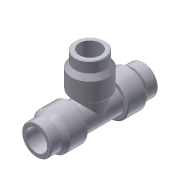
# Autodesk Inventor part: 0pvc_T_0.75
Saved by Autodesk Inventor 2016 (Build 200138000, 138)
## iProperties
Company: HERA Project
Created: 2013-06-12
Part Number: 0pvc_T_0.75
Material: PVC-Piping
Document SubType Name: Modeling
Designer: David DeBoer
Density: 1.4 g/cm^3
Description: 3/4" PVC Tee
Mass: 47.0427 g
Surface Area: 211.064 cm^2
Volume: 33.6019 cm^3
Appearance: Smooth - White
Author: David DeBoer
Title: PVC-T-0.75
Autodesk Inventor part; units mm, degrees
sketch "Sketch1" plane through (0, 0, 0) normal (0, 0, 1) x (1, 0, 0)
  circle A0 centre (0, 0) radius 14.5
  dimension "d0" = 29
  constraints: 1 centre point, 1 coincident
  measures "d0" diameter of A0
extrude "mainBody" add sketch "Sketch1" along normal mid plane 111
sketch "Sketch10" plane through (0, 0, 55.5) normal (0, 0, 1) x (1, 0, 0)
  circle A0 centre (0, 0) radius 30.1625 projected
  circle A1 centre (0, 0) radius 14.5 projected
  point P0 (0, 14.5)
  constraints: 1 vertical alignment, 1 other
ref_plane "Work Plane5" through (0, 14.5, 55.5) normal (0, 1, 0) x (-1, 0, 0)
sketch "Sketch11" plane through (0, 14.5, 55.5) normal (0, 1, 0) x (-1, 0, 0)
  circle A0 centre (0, -55.5) radius 14.5
  line L0 (14.5, 0) -> (-14.5, 0) projected
  point P0 (0, -55.5)
  dimension "d29" = 55.5
  dimension "d30" = 29
  constraints: 1 centre point
  measures "d29" distance from line of A0.centre L0
  measures "d30" diameter of A0
extrude "TBody" add sketch "Sketch11" along normal blind 40 and the other way blind 14
sketch "Sketch12" plane through (0, 54.5, 0) normal (0, 1, 0) x (1, 0, 0)
  circle A0 centre (0, 0) radius 14.5 projected
  circle A1 centre (0, 0) radius 11
  point P0 (0, 0)
  dimension "d35" = 22
  constraints: 1 centre point, 1 coincident
  measures "d35" diameter of A1
extrude "TSocket" cut sketch "Sketch12" against normal blind 39.5 contours A1
sketch "Sketch13" plane through (0, 15, 0) normal (0, 1, 0) x (1, 0, 0)
  circle A0 centre (0, 0) radius 11 projected
  circle A1 centre (0, 0) radius 10
  point P0 (0, 0)
  dimension "d39" = 20
  constraints: 1 centre point, 1 coincident
  measures "d39" diameter of A1
extrude "TTube" cut sketch "Sketch13" against normal blind 15.24 contours A1
sketch "Sketch14" plane through (0, 0, 55.5) normal (0, 0, 1) x (1, 0, 0)
  circle A0 centre (0, 0) radius 14.5 projected
  circle A1 centre (0, 0) radius 10
  dimension "d43" = 20
  constraints: 1 centre point, 1 coincident
  measures "d43" diameter of A1
extrude "mainTube" cut sketch "Sketch14" against normal blind 177.8 contours A1
sketch "Sketch15" plane through (0, 0, 55.5) normal (0, 0, 1) x (1, 0, 0)
  circle A0 centre (0, 0) radius 10 projected
  circle A1 centre (0, 0) radius 14.5 projected
  circle A2 centre (0, 0) radius 11
  dimension "d47" = 22
  constraints: 1 centre point, 1 coincident
  measures "d47" diameter of A2
extrude "mainSocket1" cut sketch "Sketch15" against normal blind 39.5 contours A2
sketch "Sketch16" plane through (0, 0, -55.5) normal (0, 0, -1) x (-1, 0, 0)
  circle A0 centre (0, 0) radius 10 projected
  circle A1 centre (0, 0) radius 14.5 projected
  circle A2 centre (0, 0) radius 11
  dimension "d51" = 22
  constraints: 1 centre point, 1 coincident
  measures "d51" diameter of A2
extrude "mainSocket2" cut sketch "Sketch16" against normal blind 39.5 contours A2
sketch "Sketch21" plane through (0, 54.5, 0) normal (0, 1, 0) x (1, 0, 0)
  circle A0 centre (0, 0) radius 11 projected
  circle A1 centre (0, 0) radius 14.5 projected
  point P0 (0, 0)
  point P1 (14.5, 0)
  constraints: 1 horizontal alignment, 1 other
ref_plane "Work Plane6" through (14.5, 54.5, 0) normal (1, 0, 0) x (0, 1, 0)
sketch "Sketch22" plane through (14.5, 54.5, 0) normal (1, 0, 0) x (0, 1, 0)
  circle A0 centre (-23, -0.01) radius 1.7314
  line L0 (0, -14.5) -> (0, 14.5) projected
  point P0 (-54.5, 0)
  dimension "d73" = 23
  constraints: 1 centre point
  measures "d73" distance from line of A0.centre L0
extrude "Extrusion18" add sketch "Sketch22" along normal blind 0.254
sketch "Sketch23" plane through (0, 54.5, 0) normal (0, 1, 0) x (1, 0, 0)
  circle A0 centre (0, 0) radius 14.5
  circle A1 centre (0, 0) radius 19
  dimension "d76" = 38
  constraints: 2 centre point, 2 coincident
  measures "d76" diameter of A1
extrude "Extrusion19" add sketch "Sketch23" against normal blind 36
sketch "Sketch24" plane through (0, 54.5, 0) normal (0, 1, 0) x (1, 0, 0)
  circle A0 centre (0, 0) radius 19
  circle A1 centre (0, 0) radius 15.5
  dimension "d79" = 31
  constraints: 2 centre point, 2 coincident
  measures "d79" diameter of A1
extrude "Extrusion20" cut sketch "Sketch24" against normal blind 11
chamfer "Chamfer1" distance 5 distance2 3.5 1 edges at (-19, 43.5, 0) measured on face at (18.754, 26.8333, 3.0478)
fillet "Fillet1" radius 1.5 1 edges at (-19, 18.5, 0)
fillet "Fillet2" radius 0.5 1 edges at (14.5, 18.5, 0)
chamfer "Chamfer2" distance 0.75 angle 45 1 edges at (-15.5, 54.5, 0)
sketch "Sketch25" plane through (0, 0, 55.5) normal (0, 0, 1) x (1, 0, 0)
  circle A0 centre (0, 0) radius 14.5
  circle A1 centre (0, 0) radius 19
  dimension "d90" = 38
  constraints: 2 centre point, 2 coincident
  measures "d90" diameter of A1
extrude "Extrusion21" add sketch "Sketch25" against normal blind 35
sketch "Sketch26" plane through (0, 0, 55.5) normal (0, 0, 1) x (1, 0, 0)
  circle A0 centre (0, 0) radius 19
  circle A1 centre (0, 0) radius 15.5
  dimension "d93" = 31
  constraints: 2 centre point, 2 coincident
  measures "d93" diameter of A1
extrude "Extrusion22" cut sketch "Sketch26" against normal blind 11
chamfer "Chamfer3" distance 5 distance2 3.5 1 edges at (-19, 0, 44.5) measured on face at (18.9384, -1.5289, 28.5)
fillet "Fillet5" radius 1.5 1 edges at (-19, 0, 20.5)
fillet "Fillet4" radius 0.5 1 edges at (-14.5, 0, 20.5)
chamfer "Chamfer4" distance 0.75 angle 45 1 edges at (-15.5, 0, 55.5)
sketch "Sketch27" plane through (0, 0, -55.5) normal (0, 0, -1) x (-1, 0, 0)
  circle A0 centre (0, 0) radius 14.5
  circle A1 centre (0, 0) radius 19
  dimension "d105" = 38
  constraints: 2 centre point, 2 coincident
  measures "d105" diameter of A1
extrude "Extrusion23" add sketch "Sketch27" against normal blind 35
sketch "Sketch28" plane through (0, 0, -55.5) normal (0, 0, -1) x (-1, 0, 0)
  circle A0 centre (0, 0) radius 19
  circle A1 centre (0, 0) radius 15.5
  dimension "d108" = 31
  constraints: 2 centre point, 2 coincident
  measures "d108" diameter of A1
extrude "Extrusion24" cut sketch "Sketch28" against normal blind 11
chamfer "Chamfer5" distance 5 distance2 3.5 1 edges at (19, 0, -44.5) measured on face at (-18.9384, -1.5289, -28.5)
fillet "Fillet6" radius 1.5 1 edges at (19, 0, -20.5)
fillet "Fillet7" radius 0.5 1 edges at (-14.5, 0, -20.5)
chamfer "Chamfer6" distance 0.75 angle 45 1 edges at (15.5, 0, -55.5)
ref_plane "Work Plane7" through (19.1, 0, 0) normal (1, 0, 0) x (0, 1, 0)
sketch "Sketch29" plane through (19.1, 0, 0) normal (1, 0, 0) x (0, 1, 0)
  circle A0 centre (30, 0) radius 1.27
  point P0 (0, 0)
  dimension "d120" = 2.54
  dimension "d121" = 30
  constraints: 1 centre point
  measures "d120" diameter of A0
  measures "d121" distance of A0.centre point (0, 0)
extrude "Extrusion25" add sketch "Sketch29" against normal up to surface
body "Solid1"
